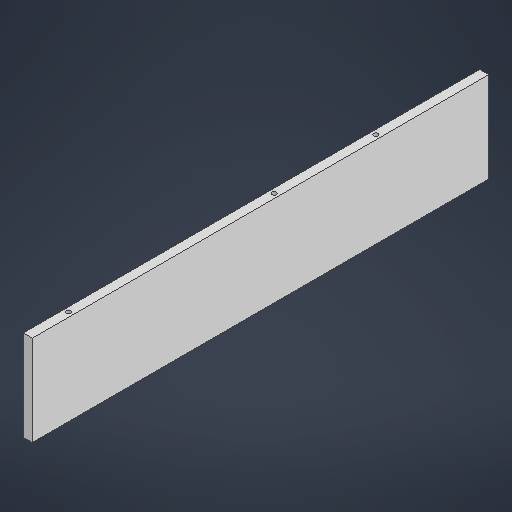
# Autodesk Inventor part: DindingRobotKananKiri
Saved by Autodesk Inventor 2026.1 (Build 301233020, 233B)
## iProperties
Created: 2025-11-08
Part Number: DindingRobotKananKiri
Material: Generic
Document SubType Name: Modeling
Designer: FrianVex
Density: 1 g/cm^3
Appearance: Default
Author: FrianVex
Autodesk Inventor part; units mm, degrees
ref_plane "YZ Plane" through (0, 0, 0) normal (1, 0, 0) x (0, 1, 0)
ref_plane "XZ Plane" through (0, 0, 0) normal (0, 1, 0) x (-1, 0, 0)
ref_plane "XY Plane" through (0, 0, 0) normal (0, 0, 1) x (1, 0, 0)
sketch "Sketch1" plane through (0, 0, 0) normal (0, 1, 0) x (-1, 0, 0)
  line L0 (2, -101) -> (-2, -101)
  line L1 (-2, -101) -> (-2, 101)
  line L2 (-2, 101) -> (2, 101)
  line L3 (2, 101) -> (2, -101)
  line L4 (2, -101) -> (-2, 101) construction
  line L5 (-2, -101) -> (2, 101) construction
  circle A0 centre (0, 83) radius 1
  circle A1 centre (0, -53) radius 1
  circle A2 centre (0, -8) radius 1
  point P0 (0, 0)
  dimension "d0" = 4
  dimension "d1" = 202
  dimension "d2" = 2
  dimension "d3" = 18
  dimension "d4" = 2
  dimension "d5" = 2
  dimension "d6" = 48
  dimension "d7" = 2
  dimension "d8" = 2
  dimension "d9" = 2
  dimension "d10" = 93
  constraints: 12 end point, 3 centre point, 2 midpoint, 2 parallel, 1 horizontal, 1 perpendicular
  measures "d0" distance of L1.end L2.end
  measures "d1" distance of L0.end L1.end
  measures "d2" diameter of A0
  measures "d3" distance from line of L2 A0.centre
  measures "d4" distance from line of L3 A0.centre
  measures "d5" diameter of A1
  measures "d6" distance from line of L0 A1.centre
  measures "d7" distance from line of L3 A1.centre
  measures "d8" diameter of A2
  measures "d9" distance from line of L3 A2.centre
  measures "d10" distance from line of L0 A2.centre
extrude "Extrusion1" add sketch "Sketch1" along normal blind 40
body "Solid1"
